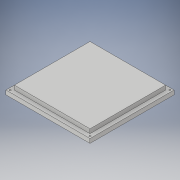
# Autodesk Inventor part: cubesat_top
Saved by Autodesk Inventor 2017 (Build 210142000, 142)
## iProperties
Created: 2016-12-15
Part Number: cubesat_top
Material: Generic
Document SubType Name: Modeling
Designer: Ali
Density: 1 g/cm^3
Appearance: Default
Author: Ali
Autodesk Inventor part; units mm, degrees
ref_plane "YZ Plane" through (0, 0, 0) normal (1, 0, 0) x (0, 1, 0)
ref_plane "XZ Plane" through (0, 0, 0) normal (0, 1, 0) x (-1, 0, 0)
ref_plane "XY Plane" through (0, 0, 0) normal (0, 0, 1) x (1, 0, 0)
sketch "Sketch1" plane through (0, 0, 0) normal (0, 1, 0) x (-1, 0, 0)
  point P0 (0, 0)
sketch "Sketch2" plane through (0, 0, 0) normal (0, 1, 0) x (-1, 0, 0)
  line L0 (50, -50) -> (-50, -50)
  line L1 (-50, -50) -> (-50, 50)
  line L2 (-50, 50) -> (50, 50)
  line L3 (50, 50) -> (50, -50)
  point P0 (0, 0)
  point P1 (0, 0)
  dimension "d0" = 100
  dimension "d1" = 100
  dimension "d3" = 50
  constraints: 8 end point, 2 parallel, 1 coincident, 1 horizontal, 1 perpendicular
  measures "d0" distance of L0.start L0.end
  measures "d1" distance of L0.end L1.end
  measures "d3" distance from line of L2 point (0, 0)
extrude "Extrusion1" add sketch "Sketch2" along normal blind 5
sketch "Sketch3" plane through (0, 5, 0) normal (0, 1, 0) x (1, 0, 0)
  circle A0 centre (-47.5, 47.5) radius 1
  line L0 (-50, 50) -> (-50, -50) projected
  line L1 (50, 50) -> (-50, 50) projected
  line L2 (50, -50) -> (50, 50) projected
  circle A1 centre (47.5, 47.5) radius 1
  line L3 (-50, -50) -> (50, -50) projected
  circle A2 centre (-47.5, -47.5) radius 1
  circle A3 centre (47.5, -47.5) radius 1
  point P0 (0, 0)
  dimension "d6" = 2.5
  dimension "d7" = 2.5
  dimension "d8" = 2
  dimension "d9" = 2.5
  dimension "d10" = 2.5
  dimension "d11" = 2.5
  dimension "d12" = 2.5
  dimension "d13" = 2.5
  dimension "d14" = 2.5
  constraints: 4 centre point, 4 coincident, 3 equal radius
  measures "d6" distance from line of L0 point (-47.5, 47.5)
  measures "d7" distance from line of L1 point (-47.5, 47.5)
  measures "d8" diameter of A0
  measures "d9" distance from line of L1 point (47.5, 47.5)
  measures "d10" distance from line of L2 point (47.5, 47.5)
  measures "d11" distance from line of L0 point (-47.5, -47.5)
  measures "d12" distance from line of L3 point (-47.5, -47.5)
  measures "d13" distance from line of L2 point (47.5, -47.5)
  measures "d14" distance from line of L3 point (47.5, -47.5)
hole "Hole1" at (-47.5062, 5, -47.5057) direction (0, -1, 0) diameter 2 end through all
hole "Hole2" at (-47.4938, 5, 47.4921) direction (0, -1, 0) diameter 2 end through all
hole "Hole3" at (47.5124, 5, 47.4796) direction (0, -1, 0) diameter 2 end through all
hole "Hole4" at (47.5, 5, -47.5) direction (0, -1, 0) diameter 2 end through all
sketch "Sketch4" plane through (0, 5, 0) normal (0, 1, 0) x (1, 0, 0)
  line L0 (-45, 45) -> (45, 45)
  line L1 (45, 45) -> (45, -45)
  line L2 (45, -45) -> (-45, -45)
  line L3 (-45, -45) -> (-45, 45)
  line L4 (50, 50) -> (50, -50) projected
  line L5 (50, 50) -> (-50, 50) projected
  line L6 (-50, 50) -> (-50, -50) projected
  line L7 (-50, -50) -> (50, -50) projected
  point P0 (0, 0)
  dimension "d49" = 5
  dimension "d50" = 5
  dimension "d51" = 5
  dimension "d52" = 5
  constraints: 8 end point, 2 parallel, 1 horizontal, 1 perpendicular
  measures "d49" distance between parallel lines of L4 L1
  measures "d50" distance between parallel lines of L5 L0
  measures "d51" distance between parallel lines of L6 L3
  measures "d52" distance between parallel lines of L7 L2
extrude "Extrusion2" add sketch "Sketch4" along normal blind 5 contours L0 L1 L2 L3
body "Solid1"
